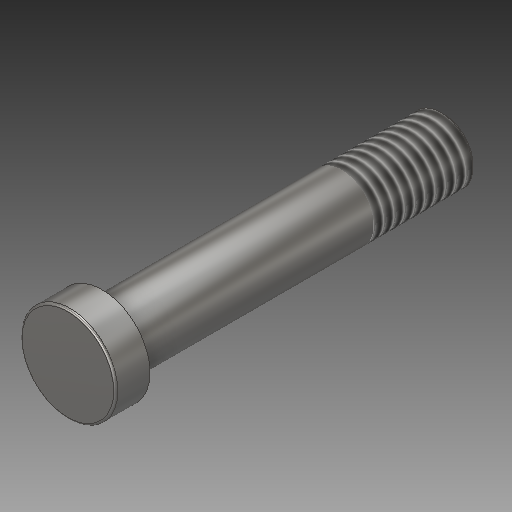
# Autodesk Inventor part: Kingpin_Bolt
Saved by Autodesk Inventor 2019 (Build 230136000, 136)
## iProperties
Created: 2020-12-09
Part Number: Kingpin_Bolt
Material: Steel, Carbon
Document SubType Name: Modeling
Designer: Anass Hamdi
Density: 7.85 g/cm^3
Appearance: Semi-Polished
Author: Anass Hamdi
Autodesk Inventor part; units mm, degrees
ref_plane "YZ Plane" through (0, 0, 0) normal (1, 0, 0) x (0, 1, 0)
ref_plane "XZ Plane" through (0, 0, 0) normal (0, 1, 0) x (-1, 0, 0)
ref_plane "XY Plane" through (0, 0, 0) normal (0, 0, 1) x (1, 0, 0)
sketch "Sketch1" plane through (0, 0, 0) normal (0, 0, 1) x (1, 0, 0)
  circle A0 centre (0, 0) radius 7
  dimension "d0" = 14
  constraints: 1 centre point, 1 coincident
  measures "d0" diameter of A0
extrude "Extrusion1" add sketch "Sketch1" along normal blind 5
sketch "Sketch2" plane through (0, 0, 0) normal (0, 0, -1) x (-1, 0, 0)
  circle A0 centre (0, 0) radius 4.7
  dimension "d3" = 9.4
  constraints: 1 centre point, 1 coincident
  measures "d3" diameter of A0
extrude "Extrusion2" add sketch "Sketch2" along normal blind 50
fillet "Fillet1" radius 0.3 1 edges at (-7, 0, 5)
thread "Thread1" size "M10x1.5" class "6g" standard "ANSI Metric M Profile" length 15
chamfer "Chamfer1" distance 0.5 angle 45 1 edges at (4.7, 0, -50)
sketch "Sketch3" plane through (0, 0, 0) normal (0, 1, 0) x (-1, 0, 0)
  ellipse E0 centre (0, -50) end of major axis (4.2, -50) minor radius 0.5 (4.2, -50) -> (0, -49.5) ccw
  line L0 (4.2, -50) -> (0, -50)
  line L1 (0, -50) -> (0, -49.5)
  point P0 (0, 0)
  constraints: 4 end point, 1 horizontal, 1 vertical, 4 other
revolve "Revolution1" cut sketch "Sketch3" angle 360 about axis through (0, 0, -50) along (0, 0, 1)
body "Solid1"
